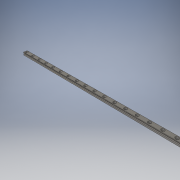
# Autodesk Inventor part: mgn9_350mm
Saved by Autodesk Inventor 2016 (Build 200138000, 138)
## iProperties
Created: 2016-06-03
Part Number: mgn9_350mm
Material: Generic
Document SubType Name: Modeling
Designer: brent
Density: 1 g/cm^3
Appearance: Steel - Polished
Author: brent
Autodesk Inventor part; units mm, degrees
ref_plane "YZ Plane" through (0, 0, 0) normal (1, 0, 0) x (0, 1, 0)
ref_plane "XZ Plane" through (0, 0, 0) normal (0, 1, 0) x (-1, 0, 0)
ref_plane "XY Plane" through (0, 0, 0) normal (0, 0, 1) x (1, 0, 0)
sketch "Sketch1" plane through (0, 0, 0) normal (1, 0, 0) x (0, 1, 0)
  line L0 (0, 0) -> (6.5, 0)
  line L1 (6.5, 0) -> (6.5, -9)
  line L2 (6.5, -9) -> (0, -9)
  line L3 (0, -9) -> (0, 0)
  dimension "d0" = 6.5
  dimension "d1" = 9
  constraints: 8 end point, 2 parallel, 1 horizontal, 1 perpendicular
  measures "d0" distance of L1.end L2.end
  measures "d1" distance of L0.end L1.end
extrude "Extrusion1" add sketch "Sketch1" along normal blind 350
sketch "Sketch2" plane through (350, 0, 0) normal (1, 0, 0) x (0, 0, -1)
  line L0 (0, 6.5) -> (0, 0) projected
  line L1 (0, 0) -> (9, 0) construction
  line L2 (9, 0) -> (9, 6.5) projected
  line L3 (9, 6.5) -> (0, 6.5) construction
  line L4 (0, 3) -> (1.25, 4.25)
  line L5 (1.25, 4.25) -> (0, 5.5)
  line L6 (9, 6.5) -> (0, 6.5) projected
  line L7 (4.5, 6.5) -> (4.5, 0) construction
  line L8 (0, 0) -> (9, 0) projected
  line L9 (9, 3) -> (7.75, 4.25)
  line L10 (7.75, 4.25) -> (9, 5.5)
  line L11 (9, 5.5) -> (9, 3)
  line L12 (9, 0) -> (9, 6.5) projected
  dimension "d4" = 3.5
  dimension "d5" = 1
  dimension "d6" = 45
  constraints: 12 end point, 3 symmetric about line, 2 midpoint, 2 point on line, 1 collinear, 1 perpendicular
  measures "d4" distance from line of L3 L4.start
  measures "d5" distance from line of L3 L5.end
  measures "d6" angle of L0 L5
extrude "Extrusion2" cut sketch "Sketch2" against normal through all contours L5 L4 L0 | L2 L9 L10
chamfer "Chamfer1" distance 0.5 angle 45 4 edges at (175, 6.5, 0) (175, 6.5, -9) (175, 4.25, -7.75) (175, 4.25, -1.25)
sketch "Sketch3" plane through (0, 6.5, -0.5) normal (0, 1, 0) x (1, 0, 0)
  line L0 (0, 8) -> (350, 8) projected
  line L1 (0, 0) -> (0, 8) projected
  line L2 (350, 0) -> (0, 0) projected
  line L3 (350, 8) -> (350, 0) projected
  line L4 (0, 4) -> (5, 4)
  circle A0 centre (5, 4) radius 1.75
  circle A1 centre (5, 4) radius 3
  point P0 (0, -0.5)
  dimension "d12" = 3.5
  dimension "d13" = 5
  dimension "d14" = 6
  constraints: 2 centre point, 2 coincident, 2 end point, 1 horizontal, 1 midpoint
  measures "d12" diameter of A0
  measures "d13" distance of L4.start L4.end
  measures "d14" diameter of A1
extrude "Extrusion3" cut sketch "Sketch3" against normal through all contours A0
extrude "Extrusion4" cut sketch "Sketch3" against normal blind 3.5 contours A1
pattern_linear "Rectangular Pattern1" count 18 spacing 20 along (1, 0, 0) of "Extrusion3", "Extrusion4"
body "Solid1"
